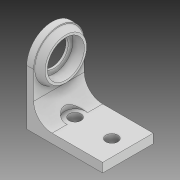
# Autodesk Inventor part: Winder_idler
Saved by Autodesk Inventor 2020 (Build 240168000, 168)
## iProperties
Created: 2021-03-13
Part Number: Winder_idler
Material: Generic
Document SubType Name: Modeling
Designer: DDeGo
Density: 1 g/cm^3
Appearance: Default
Author: DDeGo
Autodesk Inventor part; units mm, degrees
ref_plane "YZ Plane" through (0, 0, 0) normal (1, 0, 0) x (0, 1, 0)
ref_plane "XZ Plane" through (0, 0, 0) normal (0, 1, 0) x (-1, 0, 0)
ref_plane "XY Plane" through (0, 0, 0) normal (0, 0, 1) x (1, 0, 0)
sketch "Sketch3" plane through (0, 0, 0) normal (0, 0, 1) x (1, 0, 0)
  line L0 (0, 0) -> (0, 35)
  line L1 (0, 35) -> (3, 35)
  line L2 (3, 35) -> (3, 4)
  line L3 (3, 4) -> (33, 4)
  line L4 (33, 4) -> (33, 0)
  line L5 (33, 0) -> (0, 0)
  line L6 (0, 25) -> (3, 25) construction
  dimension "d0" = 10
  dimension "d1" = 25
  dimension "d2" = 30
  dimension "d3" = 4
  dimension "d4" = 3
  constraints: 14 end point, 5 perpendicular, 2 point on line, 1 horizontal, 1 vertical
  measures "d0" distance between parallel lines of L1 L6
  measures "d1" distance between parallel lines of L5 L6
  measures "d2" distance of L2.end L3.end
  measures "d3" distance between parallel lines of L5 L3
  measures "d4" distance of L0.end L1.end
extrude "Extrusion1" add sketch "Sketch3" along normal mid plane 22
sketch "Sketch4" plane through (3, 4, -11) normal (1, 0, 0) x (0, 0, -1)
  line L0 (0, 31) -> (-22, 31) construction
  line L1 (-11, 31) -> (-11, 20) construction
  circle A0 centre (-11, 20) radius 8.05
  point P0 (-11, -4)
  dimension "d7" = 11
  dimension "d8" = 16.1
  constraints: 2 end point, 1 centre point, 1 coincident, 1 midpoint, 1 vertical
  measures "d7" distance of L1.start L1.end
  measures "d8" diameter of A0
extrude "Extrusion2" cut sketch "Sketch4" against normal through all
fillet "Fillet3" radius 8 1 edges at (3, 4, 0)
sketch "Sketch5" plane through (3, 4, -11) normal (0, 1, 0) x (1, 0, 0)
  line L0 (30, 0) -> (30, -22) construction
  line L1 (30, -11) -> (0, -11) construction
  line L2 (0, 0) -> (0, -22) construction
  circle A0 centre (7, -11) radius 2.6
  circle A1 centre (23, -11) radius 2.6
  point P0 (-3, -11)
  dimension "d11" = 7
  dimension "d12" = 7
  dimension "d13" = 5.2
  constraints: 2 centre point, 2 end point, 2 midpoint, 2 point on line, 1 equal radius
  measures "d11" distance from line of L0 A1.centre
  measures "d12" distance from line of L2 A0.centre
  measures "d13" diameter of A0
extrude "Extrusion3" cut sketch "Sketch5" along normal mid plane 24.75
sketch "Sketch6" plane through (0, 0, 0) normal (0, 0, 1) x (1, 0, 0)
  line L0 (3, 15.95) -> (0, 15.95) construction
  line L1 (0, 15.95) -> (0, 17.95)
  line L2 (0, 17.95) -> (1, 17.95)
  line L3 (1, 17.95) -> (1, 15.95)
  line L4 (0, 15.95) -> (0, 32.05) construction
  line L5 (1, 15.95) -> (0, 15.95)
  line L6 (3, 32.05) -> (3, 15.95) construction
  line L7 (3, 15.95) -> (6, 15.95)
  line L8 (6, 15.95) -> (6, 14.95)
  line L9 (6, 14.95) -> (3, 13.45)
  line L10 (3, 13.45) -> (3, 15.95)
  line L11 (0, 24) -> (3, 24) construction
  point P0 (0, 0)
  dimension "d16" = 1
  dimension "d17" = 2
  dimension "d18" = 5
  dimension "d19" = 2.5
  dimension "d20" = 1
  constraints: 18 end point, 5 perpendicular, 2 midpoint, 1 horizontal, 1 point on line, 1 vertical
  measures "d16" distance between parallel lines of L1 L3
  measures "d17" distance of L2.end L3.end
  measures "d18" distance between parallel lines of L8 L3
  measures "d19" distance of L9.end L0.start
  measures "d20" distance of L7.end L8.end
revolve "Revolution1" add sketch "Sketch6" angle 360 about axis through (0, 24, 0) along (1, 0, 0)
fillet "Fillet1" radius 11 2 edges at (1.5, 35, 11) (1.5, 35, -11)
sketch "Sketch11" plane through (33, 4, 11) normal (0, 1, 0) x (1, 0, 0)
  circle A0 centre (-23, 11) radius 2.6 projected
  circle A1 centre (-23, 11) radius 4.5
  point P0 (-33, 11)
  dimension "d42" = 9
  constraints: 1 centre point, 1 coincident
  measures "d42" diameter of A1
extrude "Extrusion8" cut sketch "Sketch11" along normal blind 5 contours A0 | A1
body "Solid1"
